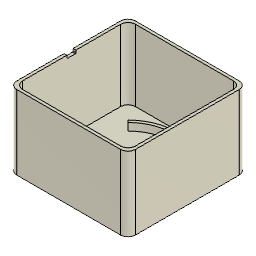
box (Autodesk Fusion 360 design; units mm, degrees)
part number: 2025-11-17-16-15-39-081
Autodesk Fusion 360 part; units mm, degrees
sketch "Sketch1" plane through (0, 0, 0) normal (0, 0, 1) x (1, 0, 0)
box "BoxPrimitive1" add length 80 width 80 height 50 placed x (0, 1, 0) y (-1, 0, 0) z (0, 0, 1) at (72, 0, 0)
sketch "Sketch3" plane through (0, 0, 50) normal (0, 0, 1) x (-1, 0, 0)
  line L0 (-72, -80) -> (8, -80)
  line L1 (8, -80) -> (8, 0)
  line L2 (8, 0) -> (-72, 0)
  line L3 (-72, 0) -> (-72, -80)
  line L4 (8, 0) -> (-72, 0)
  line L5 (-72, 0) -> (-72, -80)
  line L6 (-72, -80) -> (8, -80)
  line L7 (8, -80) -> (8, 0)
  line L8 (8, 0) -> (-72, -80) construction
  line L9 (-72, 0) -> (8, -80) construction
  line L10 (6, -78) -> (-70, -78)
  line L11 (-70, -78) -> (-70, -2)
  line L12 (-70, -2) -> (6, -2)
  line L13 (6, -2) -> (6, -78)
  line L14 (6, -78) -> (-70, -2) construction
  line L15 (-70, -78) -> (6, -2) construction
  line L16 (-32, 0) -> (-32, -80)
  line L17 (8, -40) -> (-72, -40)
  point P0 (-32, -40)
  point P1 (-32, -40)
  dimension "d14" = 80
  dimension "d17" = 76
  constraint horizontal L4
  constraint perpendicular L4 L5
  constraint parallel L4 L6
  constraint parallel L5 L7
  constraint coincident L8 P1
  constraint coincident L9 P1
  constraint horizontal L10
  constraint perpendicular L10 L11
  constraint parallel L10 L12
  constraint parallel L11 L13
  constraint coincident L14 P1
  constraint coincident L15 P1
  constraint coincident P1 P0
  constraint midpoint L4 L16.start
  constraint midpoint L6 L16.end
  constraint midpoint L7 L17.start
  constraint midpoint L3 L17.end
  measures "d14" distance of L0.start L0.end
  measures "d17" distance of L10.end L11.end
extrude "Extrude1" cut sketch "Sketch3" against normal blind 48 contours L10 L13 L16 L17 | L10 L11 L16 L17 | L11 L12 L16 L17 | L12 L13 L16 L17
sketch "Sketch4" plane through (0, 0, 0) normal (1, 0, 0) x (0, 1, 0)
  line L0 (0, 50) -> (80, 50)
  line L1 (43, 48) -> (37, 48)
  line L2 (37, 48) -> (37, 50)
  line L3 (43, 50) -> (43, 48)
  line L4 (43, 48) -> (40, 50) construction
  line L5 (37, 48) -> (40, 50) construction
  constraint horizontal L0
  constraint horizontal L1
  constraint perpendicular L1 L2
  constraint parallel L2 L3
  constraint midpoint L0 L4.end
  constraint coincident L0 L2.end
  constraint coincident L0 L3.start
extrude "Extrude2" cut sketch "Sketch4" against normal blind 10
fillet "Fillet1" radius 5 4 edges at (-6, 78, 26) (-6, 2, 26) (70, 2, 26) (70, 78, 26)
sketch "Sketch6" plane through (0, 0, 0) normal (0, -1, 0) x (1, 0, 0)
  line L0 (-8, 50) -> (-8, 0)
  line L1 (-8, 0) -> (72, 0)
  line L2 (72, 0) -> (72, 50)
  line L3 (72, 50) -> (-8, 50)
ref_plane "WorkPlane1" through (0, 40, 0) normal (0, -1, 0) x (1, 0, 0)
sketch "Sketch7" plane through (0, 40, 0) normal (0, -1, 0) x (-1, 0, 0)
fillet "Fillet2" radius 0.5 2 edges at (-7, 37, 48) (-7, 43, 48)
sketch "Sketch8" plane through (0, 0, 2) normal (0, 0, 1) x (-1, 0, 0)
  circle A0 centre (-32, -40) radius 30
  circle A1 centre (-32, -40) radius 32
  line L0 (-32, -40) -> (-32, -7)
  line L1 (-32, -40) -> (-32, -72)
  line L2 (-32, -40) -> (0, -40)
  line L3 (-32, -40) -> (-64, -40)
  line L4 (-32, -40) -> (-9.3726, -62.6274)
  line L5 (-32, -40) -> (-54.6505, -62.6505)
  line L6 (-32, -40) -> (-64.0327, -40) construction
  line L7 (-32, -40) -> (-9.3726, -17.3726)
  line L8 (-32, -40) -> (0, -40) construction
  line L9 (-32, -40) -> (-54.6274, -17.3726)
  line L10 (-32, -40) -> (-64, -40) construction
  arc A2 (-70, -73) -> (-65, -78) centre (-65, -73) ccw
  line L11 (-65, -78) -> (1, -78)
  arc A3 (1, -78) -> (6, -73) centre (1, -73) ccw
  line L12 (6, -73) -> (6, -7)
  arc A4 (6, -7) -> (1, -2) centre (1, -7) ccw
  line L13 (1, -2) -> (-65, -2)
  arc A5 (-65, -2) -> (-70, -7) centre (-65, -7) ccw
  line L14 (-70, -7) -> (-70, -73)
  dimension "d29" = 45
  dimension "d30" = 45
  dimension "d31" = 45
  dimension "d32" = 45
  constraint concentric A0 A1
  constraint coincident A0.centre A1.centre
  constraint coincident A1 L1.end
  constraint parallel L0 L1
  constraint coincident A1 L2.end
  constraint perpendicular L1 L2
  constraint coincident A1 L3.end
  constraint perpendicular L0 L3
  constraint coincident A1 L4.end
  constraint horizontal L6
  constraint horizontal L8
  constraint horizontal L10
  constraint coincident A1 L9.end
  measures "d29" angle of L3 L4
  measures "d30" angle of L5 L6
  measures "d31" angle of L7 L8
  measures "d32" angle of L9 L10
extrude "Extrude3" add sketch "Sketch8" along normal blind 5 contours A0 A1 L0 L7 | A0 A1 L1 L4 | A0 A1 L0 L9 | A0 A1 L1 L5
fillet "Fillet3" radius 5 4 edges at (72, 80, 25) (72, 0, 25) (-8, 80, 25) (-8, 0, 25)
